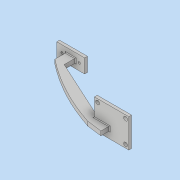
# Autodesk Inventor part: 左侧外部机械
Saved by Autodesk Inventor 2019 (Build 230136000, 136)
## iProperties
Created: 2020-12-07
Part Number: 左侧外部机械
Material: Generic
Document SubType Name: Modeling
Designer: Wang Hua
Density: 1 g/cm^3
Appearance: Default
Author: Wang Hua
Autodesk Inventor part; units mm, degrees
ref_plane "YZ Plane" through (0, 0, 0) normal (1, 0, 0) x (0, 1, 0)
ref_plane "XZ Plane" through (0, 0, 0) normal (0, 1, 0) x (-1, 0, 0)
ref_plane "XY Plane" through (0, 0, 0) normal (0, 0, 1) x (1, 0, 0)
sketch "草图1" plane through (0, 0, 0) normal (0, 0, 1) x (1, 0, 0)
  line L0 (18.5, -15.5) -> (-18.5, -15.5)
  line L1 (-18.5, -15.5) -> (-18.5, 15.5)
  line L2 (-18.5, 15.5) -> (18.5, 15.5)
  line L3 (18.5, 15.5) -> (18.5, -15.5)
  line L4 (18.5, -15.5) -> (-18.5, 15.5) construction
  line L5 (-18.5, -15.5) -> (18.5, 15.5) construction
  line L6 (0, 0) -> (0, 18.5742) construction
  line L7 (0, 0) -> (-42.7004, 0) construction
  point P0 (-15, 12)
  point P1 (15, 12)
  point P2 (-15, -12)
  point P3 (15, -12)
  dimension "d0" = 31
  dimension "d1" = 37
  dimension "d2" = 3.5
  dimension "d3" = 3.5
  dimension "d4" = 30
  constraints: 16 end point, 3 symmetric about line, 2 horizontal, 2 midpoint, 2 parallel, 1 perpendicular, 1 vertical
  measures "d0" distance of L0.end L1.end
  measures "d1" distance of L0.start L0.end
  measures "d2" distance from line of L2 point (-15, 12)
  measures "d3" distance from line of L1 point (-15, 12)
  measures "d4" distance of point (15, 12) point (-15, 12)
extrude "拉伸1" add sketch "草图1" along normal blind 3
hole "孔1" at (-15, 12, 0) at (15, 12, 0) at (-15, -12, 0) at (15, -12, 0) direction (0, 0, 1) diameter 4.2 end through all
ref_plane "工作平面1" through (-18.5, 6, 0) normal (0, -1, 0) x (1, 0, 0)
sketch "草图2" plane through (-18.5, 6, 0) normal (0, -1, 0) x (1, 0, 0)
  line L0 (0, 0) -> (37, 0) construction
  line L1 (0, 0) -> (0, 3) construction
  line L2 (37, 3) -> (0, 3) construction
  line L3 (37, 0) -> (37, 3) construction
  line L4 (0, 0) -> (37, 0) projected
  line L5 (16, 0) -> (16, 12)
  line L6 (0, 0) -> (0, 3) projected
  line L7 (0, 0) -> (0, 3)
  line L8 (-75.5, -30) -> (-65.5, -30)
  line L9 (-65.5, -30) -> (0, 0)
  line L10 (0, 10) -> (16, 12)
  line L11 (0, 0) -> (16, 0)
  line L12 (0, 0) -> (16, 0)
  arc A0 (0, 10) -> (-75.5, -30) centre (75.1487, -223.0963) ccw
  point P0 (18.5, 0)
  dimension "d15" = 10
  dimension "d16" = 30
  dimension "d17" = 65.5
  dimension "d19" = 12
  dimension "d20" = 16
  dimension "d40" = 10
  dimension "d60" = 244.9106
  constraints: 14 end point, 2 collinear, 2 point on circle, 2 point on line, 2 vertical, 1 centre point, 1 parallel, 1 perpendicular
  measures "d15" distance of L8.start L8.end
  measures "d16" distance between parallel lines of L0 L8
  measures "d17" horizontal distance of L0.start L8.end
  measures "d19" distance of L5.start L5.end
  measures "d20" horizontal distance of L5.end L10.start
  measures "d40" distance of L0.start L10.start
  measures "d60" radius of A0
extrude "拉伸2" add sketch "草图2" along normal mid plane 4.5
sketch "草图3" plane through (-84, 3.75, -30) normal (0, 0, -1) x (-1, 0, 0)
  line L0 (0, 4.5) -> (0, 0) construction
  line L1 (10, 0) -> (0, 0) construction
  line L2 (10, 4.5) -> (10, 0) construction
  line L3 (0, 4.5) -> (10, 4.5) construction
  line L4 (19, 10) -> (-11, 10)
  line L5 (-11, 10) -> (-11, -5)
  line L6 (-11, -5) -> (19, -5)
  line L7 (19, -5) -> (19, 10)
  line L8 (19, 10) -> (-11, -5) construction
  line L9 (-11, 10) -> (19, -5) construction
  point P0 (-84, -3.75)
  point P1 (4, 2.5)
  point P2 (13.3, 2.5)
  point P3 (-5.3, 2.5)
  dimension "d24" = 30
  dimension "d25" = 9.3
  dimension "d26" = 9.3
  dimension "d27" = 15
  dimension "d28" = 2.5
  dimension "d29" = 4
  constraints: 12 end point, 2 midpoint, 2 parallel, 1 horizontal, 1 perpendicular
  measures "d24" horizontal distance of L4.end L6.end
  measures "d25" distance of point (13.3, 2.5) point (4, 2.5)
  measures "d26" distance of point (4, 2.5) point (-5.3, 2.5)
  measures "d27" distance of L6.end L4.start
  measures "d28" distance from line of L1 point (4, 2.5)
  measures "d29" distance from line of L0 point (4, 2.5)
sketch "草图4" plane through (-84, 3.75, -30) normal (0, 0, -1) x (-1, 0, 0)
  line L0 (0, 4.5) -> (0, 0) projected
  line L1 (10, 0) -> (0, 0) projected
  line L2 (10, 4.5) -> (10, 0) projected
  line L3 (0, 4.5) -> (10, 4.5) projected
  point P0 (-84, -3.75)
extrude "拉伸4" add sketch "草图4" along normal blind 15
sketch "草图5" plane through (-84, 3.75, -45) normal (0, 0, -1) x (-1, 0, 0)
  line L0 (-10, 9.75) -> (20, 9.75)
  line L1 (20, 9.75) -> (20, -5.25)
  line L2 (20, -5.25) -> (-10, -5.25)
  line L3 (-10, -5.25) -> (-10, 9.75)
  line L4 (-10, 9.75) -> (20, -5.25) construction
  line L5 (20, 9.75) -> (-10, -5.25) construction
  line L6 (0, 4.5) -> (0, 0) projected
  line L7 (0, 0) -> (10, 0) projected
  point P0 (-84, -3.75)
  point P1 (5, 2.25)
  point P2 (14.3, 2.25)
  point P3 (-4.3, 2.25)
  dimension "d43" = 30
  dimension "d44" = 15
  dimension "d45" = 5
  dimension "d46" = 2.25
  dimension "d47" = 9.3
  dimension "d48" = 9.3
  dimension "d58" = 10
  constraints: 12 end point, 2 midpoint, 2 parallel, 1 horizontal, 1 perpendicular
  measures "d43" distance of L1.end L2.end
  measures "d44" distance of L0.end L1.end
  measures "d45" distance from line of L6 point (5, 2.25)
  measures "d46" distance from line of L7 point (5, 2.25)
  measures "d47" distance of point (5, 2.25) point (-4.3, 2.25)
  measures "d48" distance of point (5, 2.25) point (14.3, 2.25)
  measures "d58" distance of L6.end L7.end
extrude "拉伸5" add sketch "草图5" against normal blind 3
hole "孔3" at (-98.3, 6, -45) at (-79.7, 6, -45) direction (0, 0, 1) diameter 2.4 depth 3 tip angle 118
ref_plane "工作平面2" through (-18.5, 0, 0) normal (0, -1, 0) x (1, 0, 0)
mirror "镜像1" about plane through (-18.5, 0, 0) normal (0, -1, 0) remove original yes
fillet "圆角1" radius 0.8 9 edges at (-89, -8.25, -42) (-84, -6, -42) (-10.5, -8.25, 3) (-2.5, -6, 3) (-10.5, -3.75, 3) (-18.5, -3.75, 1.5) (-18.5, -8.25, 1.5) (-94, -6, -42) (-89, -3.75, -42)
